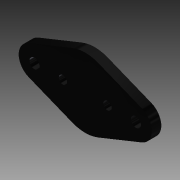
# Autodesk Inventor part: Pneumatic Mounting Plate
Saved by Autodesk Inventor 2013 (Build 170138000, 138)
## iProperties
Created: 2013-06-08
Part Number: Pneumatic Mounting Plate
Material: Generic
Document SubType Name: Modeling
Designer: mvarma
Density: 1 g/cm^3
Author: mvarma
Autodesk Inventor part; units mm, degrees
ref_plane "YZ Plane" through (0, 0, 0) normal (1, 0, 0) x (0, 1, 0)
ref_plane "XZ Plane" through (0, 0, 0) normal (0, 1, 0) x (-1, 0, 0)
ref_plane "XY Plane" through (0, 0, 0) normal (0, 0, 1) x (1, 0, 0)
sketch "Sketch1" plane through (0, 0, 0) normal (0, 0, 1) x (1, 0, 0)
  arc A0 (0, 14.224) -> (0, -14.224) centre (0, 0) ccw construction
  arc A1 (0, 17.4307) -> (0, -17.4308) centre (0, 0) ccw
  line L0 (0, 0) -> (-25.4, 0)
  circle A2 centre (-25.4, 0) radius 4.7625 construction
  line L1 (0, 14.224) -> (0, -14.224)
  circle A3 centre (-25.4, 0) radius 7.9692
  line L2 (0, 14.224) -> (0, 17.4307)
  line L3 (0, -14.224) -> (0, -17.4308)
  line L4 (-28.3685, 7.3957) -> (-6.493, 16.1763)
  line L5 (-28.3685, -7.3957) -> (-6.493, -16.1763)
  point P0 (-11.176, 0)
  dimension "d0" = 28.448
  dimension "d2" = 25.4
  dimension "d3" = 9.525
  dimension "d6" = 3.2067
  dimension "d7" = 3.2067
  dimension "d8" = 11.176
  constraints: 12 end point, 8 point on circle, 5 tangent, 4 centre point, 4 coincident, 2 collinear, 1 horizontal, 1 midpoint, 1 point on line, 1 vertical
  measures "d0" diameter of A0
  measures "d2" distance of L0.start L0.end
  measures "d3" diameter of A2
  measures "d6" radial gap between concentric circles of A2 A3
  measures "d7" radial gap between concentric circles of A1 A0
  measures "d8" distance from line of L1 point (-11.176, 0)
extrude "Extrusion1" add sketch "Sketch1" along normal blind 4.7625
hole "Hole1" at (-25.4, 0, 0) direction (0, 0, 1) diameter 5.1054 end through all clearance for "Socket Head Cap Screw" size "#10" standard "Ansi Unified Screw Threads"
hole "Hole2" at (-11.176, 0, 0) direction (0, 0, 1) diameter 4.2164 end through all
mirror "Mirror1" about plane through (0, -17.4308, 0) normal (1, 0, 0)
equation "\"d6\" = d7"
body "Solid1"
